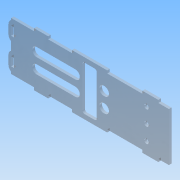
# Autodesk Inventor part: Top_plate2
Saved by Autodesk Inventor 2016 (Build 200138000, 138)
## iProperties
Created: 2015-06-18
Part Number: Top_plate2
Material: Generic
Document SubType Name: Modeling
Designer: Openlab
Density: 1 g/cm^3
Appearance: Polycarbonate - Clear
Author: Openlab
Autodesk Inventor part; units mm, degrees
ref_plane "YZ Plane" through (0, 0, 0) normal (1, 0, 0) x (0, 1, 0)
ref_plane "XZ Plane" through (0, 0, 0) normal (0, 1, 0) x (-1, 0, 0)
ref_plane "XY Plane" through (0, 0, 0) normal (0, 0, 1) x (1, 0, 0)
sketch "Sketch1" plane through (0, 0, 0) normal (0, 1, 0) x (-1, 0, 0)
  line L0 (37.25, -2.25) -> (24.75, -2.25) construction
  line L1 (24.75, -2.25) -> (24.75, -14.75) construction
  line L2 (24.75, -14.75) -> (37.25, -14.75) construction
  line L3 (37.25, -14.75) -> (37.25, -2.25) construction
  line L4 (56.9183, -8.5) -> (8.3915, -8.5) construction
  line L5 (0, -17) -> (105, -17) construction
  line L6 (0, 0) -> (0, -51) construction
  line L7 (0, -34) -> (105, -34) construction
  line L8 (105, -51) -> (105, 0) construction
  line L9 (31, 19) -> (31, -51) construction
  line L10 (56.8064, -25.5) -> (17, -25.5) construction
  line L11 (24.75, -19.25) -> (24.75, -31.75) construction
  line L12 (37.25, -19.25) -> (24.75, -19.25) construction
  line L13 (37.25, -31.75) -> (37.25, -19.25) construction
  line L14 (24.75, -31.75) -> (37.25, -31.75) construction
  line L15 (24.75, -36.25) -> (24.75, -48.75) construction
  line L16 (37.25, -36.25) -> (24.75, -36.25) construction
  line L17 (37.25, -48.75) -> (37.25, -36.25) construction
  line L18 (24.75, -48.75) -> (37.25, -48.75) construction
  line L19 (56.3008, -42.5) -> (16.5498, -42.5) construction
  arc A0 (47.05, -12) -> (47.05, -22) centre (47.05, -17) ccw
  arc A1 (91, -22) -> (91, -12) centre (91, -17) ccw
  arc A2 (47.05, -29) -> (47.05, -39) centre (47.05, -34) ccw
  arc A3 (91, -39) -> (91, -29) centre (91, -34) ccw
  line L20 (47.05, -12) -> (91, -12)
  line L21 (47.05, -22) -> (91, -22)
  line L22 (47.05, -29) -> (91, -29)
  line L23 (47.05, -39) -> (91, -39)
  arc A4 (14.95, -39) -> (14.95, -29) centre (14.95, -34) ccw
  line L24 (103.5, -49.5) -> (103.5, -1.5) construction
  line L25 (1.5, -1.5) -> (1.5, -49.5) construction
  arc A5 (14, -29) -> (14, -39) centre (14, -34) ccw
  arc A6 (14, -12) -> (14, -22) centre (14, -17) ccw
  line L26 (14.95, -39) -> (14, -39)
  line L27 (14, -29) -> (14.95, -29)
  line L28 (14, -22) -> (14.95, -22)
  line L29 (14.95, -12) -> (14, -12)
  arc A7 (14.95, -22) -> (14.95, -12) centre (14.95, -17) ccw
  arc A8 (96.5, -51) -> (93, -47.5) centre (93, -51) ccw construction
  arc A9 (47.05, -47.5) -> (43.55, -51) centre (47.05, -51) ccw construction
  arc A10 (97.7697, -49.5) -> (93, -46) centre (93, -51) ccw construction
  line L30 (93, -46) -> (47.05, -46) construction
  line L31 (96.5, -51) -> (105, -51) construction
  line L32 (93, -47.5) -> (47.05, -47.5) construction
  line L33 (105, -49.5) -> (97.7697, -49.5) construction
  arc A11 (47.05, -46) -> (42.2803, -49.5) centre (47.05, -51) ccw construction
  arc A12 (42.2803, -1.5) -> (47.05, -5) centre (47.05, 0) ccw construction
  arc A13 (43.55, 0) -> (47.05, -3.5) centre (47.05, 0) ccw construction
  line L34 (93, -3.5) -> (47.05, -3.5) construction
  line L35 (93, -5) -> (47.05, -5) construction
  line L36 (97.7697, -1.5) -> (105, -1.5) construction
  line L37 (105, 0) -> (96.5, 0) construction
  arc A14 (93, -3.5) -> (96.5, 0) centre (93, 0) ccw construction
  arc A15 (93, -5) -> (97.7697, -1.5) centre (93, 0) ccw construction
  arc A16 (16.65, -51) -> (13.15, -47.5) centre (13.15, -51) ccw construction
  arc A17 (12, -47.5) -> (8.5, -51) centre (12, -51) ccw construction
  line L38 (13.15, -46) -> (12, -46) construction
  line L39 (13.15, -47.5) -> (12, -47.5) construction
  arc A18 (12, -46) -> (7.2303, -49.5) centre (12, -51) ccw construction
  arc A19 (17.9197, -49.5) -> (13.15, -46) centre (13.15, -51) ccw construction
  line L40 (42.2803, -49.5) -> (17.9197, -49.5) construction
  line L41 (7.2303, -49.5) -> (0, -49.5) construction
  line L42 (0, -51) -> (8.5, -51) construction
  line L43 (16.65, -51) -> (43.55, -51) construction
  line L44 (13.15, -5) -> (12, -5) construction
  line L45 (13.15, -3.5) -> (12, -3.5) construction
  arc A20 (8.5, 0) -> (12, -3.5) centre (12, 0) ccw construction
  arc A21 (13.15, -3.5) -> (16.65, 0) centre (13.15, 0) ccw construction
  arc A22 (7.2303, -1.5) -> (12, -5) centre (12, 0) ccw construction
  arc A23 (13.15, -5) -> (17.9197, -1.5) centre (13.15, 0) ccw construction
  line L46 (43.55, 0) -> (16.65, 0) construction
  line L47 (8.5, 0) -> (0, 0) construction
  line L48 (0, -1.5) -> (7.2303, -1.5) construction
  line L49 (17.9197, -1.5) -> (42.2803, -1.5) construction
  arc A24 (39.25, -2.75) -> (36.75, -0.25) centre (36.75, -2.75) ccw
  arc A25 (25.25, -0.25) -> (22.75, -2.75) centre (25.25, -2.75) ccw
  arc A26 (36.75, -50.75) -> (39.25, -48.25) centre (36.75, -48.25) ccw
  arc A27 (22.75, -48.25) -> (25.25, -50.75) centre (25.25, -48.25) ccw
  line L50 (39.25, -2.75) -> (39.25, -48.25)
  line L51 (36.75, -0.25) -> (25.25, -0.25)
  line L52 (22.75, -2.75) -> (22.75, -48.25)
  line L53 (25.25, -50.75) -> (36.75, -50.75)
  line L54 (51, -56) -> (51, -53)
  line L55 (11, -56) -> (11, -53)
  line L56 (78, -56) -> (78, -53)
  line L57 (94, -53) -> (94, -56)
  line L58 (-47, -56) -> (-47, -53)
  line L59 (94, 2) -> (94, 5)
  line L60 (78, 2) -> (78, 5)
  line L61 (51, 2) -> (51, 5)
  line L62 (11, 2) -> (11, 5)
  line L63 (-47, 2) -> (-47, 5)
  line L64 (-47, -53) -> (-59, -53)
  line L65 (-29, -53) -> (11, -53)
  line L66 (51, -53) -> (78, -53)
  line L67 (94, -53) -> (120, -53)
  line L68 (120, 2) -> (94, 2)
  line L69 (78, 2) -> (51, 2)
  line L70 (11, 2) -> (-29, 2)
  line L71 (-47, 2) -> (-59, 2)
  line L72 (-29, -53) -> (-29, -56)
  line L73 (-29, 5) -> (-29, 2)
  circle A28 centre (-33.5, -42.5) radius 2.5
  circle A29 centre (-33.5, -25.5) radius 2.5
  circle A30 centre (-33.5, -8.5) radius 2.5
  line L74 (51, 5) -> (11, 5)
  line L75 (94, 5) -> (78, 5)
  line L76 (-29, 5) -> (-47, 5)
  line L77 (94, -56) -> (78, -56)
  line L78 (51, -56) -> (11, -56)
  line L79 (-29, -56) -> (-47, -56)
  line L80 (120, -5.5) -> (116.8, -5.5)
  line L81 (116.8, -5.5) -> (116.8, -15.5)
  line L82 (116.8, -15.5) -> (120, -15.5)
  line L83 (120, -15.5) -> (120, -5.5)
  line L84 (120, -35.5) -> (116.8, -35.5)
  line L85 (116.8, -35.5) -> (116.8, -45.5)
  line L86 (116.8, -45.5) -> (120, -45.5)
  line L87 (120, -45.5) -> (120, -35.5)
  arc A31 (120, -20.8104) -> (123, -15.5) centre (116.8, -15.5) ccw
  line L88 (120, -20.8104) -> (120, -30.1896)
  arc A32 (123, -35.5) -> (120, -30.1896) centre (116.8, -35.5) ccw
  line L89 (123, -5.5) -> (123, -15.5)
  line L90 (123, -35.5) -> (123, -45.5)
  arc A33 (123, -5.5) -> (120, -0.1896) centre (116.8, -5.5) ccw
  line L91 (120, -0.1896) -> (120, 2)
  arc A34 (120, -50.8104) -> (123, -45.5) centre (116.8, -45.5) ccw
  line L92 (120, -50.8104) -> (120, -53)
  line L93 (-59, 2) -> (-59, -53)
  point P0 (31, -8.5)
  point P1 (31, -42.5)
  point P2 (31, -25.5)
  dimension "d0" = 12.5
  dimension "d1" = 12.5
  dimension "d2" = 17
  dimension "d3" = 31
  dimension "d4" = 105
  dimension "d5" = 17
  dimension "d6" = 17
  dimension "d7" = 10
  dimension "d8" = 1.5
  dimension "d9" = 1.5
  dimension "d10" = 5
  dimension "d11" = 1.5
  dimension "d12" = 1.5
  dimension "d13" = 1.5
  dimension "d14" = 17
  dimension "d15" = 17
  dimension "d16" = 12
  dimension "d17" = 14
  dimension "d19" = 11.6
  dimension "d21" = 12
  dimension "d38" = 40
  dimension "d39" = 27
  dimension "d40" = 16
  dimension "d56" = 3
  dimension "d64" = 14
  dimension "d65" = 16.05
  dimension "d66" = 10.5
  dimension "d67" = 2
  dimension "d109" = 5
  dimension "d118" = 40
  dimension "d120" = 18
  dimension "d131" = 10
  dimension "d132" = 3.2
  dimension "d134" = 20
  dimension "d136" = 3
  dimension "d138" = 26
  dimension "d140" = 12
  dimension "d141" = 25.5
  dimension "d142" = 2.5
  dimension "d143" = 2
  dimension "d144" = 2
  dimension "d145" = 16.05
  constraints: 189 end point, 64 point on circle, 36 collinear, 36 tangent, 35 centre point, 31 point on line, 27 equal radius, 20 parallel, 20 perpendicular, 15 horizontal, 14 coincident, 13 vertical alignment, 9 horizontal alignment, 5 equal length, 5 vertical, 13 other
  measures "d0" distance of L2.end L1.end
  measures "d1" distance of L0.end L1.end
  measures "d2" distance between parallel lines of L10 L4
  measures "d3" distance between parallel lines of L6 L9
  measures "d4" distance between parallel lines of L6 L8
  measures "d5" distance between parallel lines of L19 L10
  measures "d6" distance between parallel lines of L5 L7
  measures "d7" diameter of A0
  measures "d8" distance between parallel lines of L6 L25
  measures "d9" distance between parallel lines of L8 L24
  measures "d10" radius of A4
  measures "d11" radial gap between concentric circles of A8 A10
  measures "d12" distance between parallel lines of L37 L36
  measures "d13" distance between parallel lines of L41 L42
  measures "d14" distance between parallel lines of L7 L42
  measures "d15" distance between parallel lines of L47 L5
  measures "d16" distance from line of A8.centre L8
  measures "d17" distance from line of L8 A3.centre
  measures "d19" distance from line of A19.centre L15
  measures "d21" distance from line of L6 A22.centre
  measures "d38" distance between parallel lines of L55 L54
  measures "d39" distance between parallel lines of L56 L54
  measures "d40" distance between parallel lines of L56 L57
  measures "d56" distance of L60.start L60.end
  measures "d64" distance of L5.start A6.centre
  measures "d65" distance from line of L9 A11.centre
  measures "d66" distance between parallel lines of L65 L19
  measures "d67" distance between parallel lines of L31 L67
  measures "d109" diameter of A28
  measures "d118" distance between parallel lines of L72 L55
  measures "d120" distance of L72.end L58.start
  measures "d131" distance of L80.end L81.end
  measures "d132" distance of L80.start L80.end
  measures "d134" distance between parallel lines of L84 L82
  measures "d136" distance between parallel lines of L90 L87
  measures "d138" distance between parallel lines of L57 L92
  measures "d140" distance between parallel lines of L93 L58
  measures "d141" distance from line of L93 A28.centre
  measures "d142" radius of A27
  measures "d143" distance between parallel lines of L52 L1
  measures "d144" distance between parallel lines of L51 L0
  measures "d145" distance from line of A4.centre L9
extrude "Extrusion2" add sketch "Sketch1" along normal blind 3
body "Solid2"
